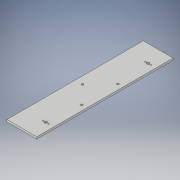
# Autodesk Inventor part: ChassisSideplate10
Saved by Autodesk Inventor 2019 (Build 230136000, 136)
## iProperties
Created: 2019-10-11
Part Number: ChassisSideplate10
Material: Generic
Document SubType Name: Modeling
Designer: shrey
Density: 1 g/cm^3
Appearance: Default
Author: shrey
Autodesk Inventor part; units mm, degrees
ref_plane "YZ Plane" through (0, 0, 0) normal (1, 0, 0) x (0, 1, 0)
ref_plane "XZ Plane" through (0, 0, 0) normal (0, 1, 0) x (-1, 0, 0)
ref_plane "XY Plane" through (0, 0, 0) normal (0, 0, 1) x (1, 0, 0)
sketch "Sketch1" plane through (0, 0, 0) normal (0, 1, 0) x (-1, 0, 0)
  line L0 (44.45, 203.2) -> (-44.45, 203.2)
  line L1 (-44.45, 203.2) -> (-44.45, -203.2)
  line L2 (-44.45, -203.2) -> (44.45, -203.2)
  line L3 (44.45, -203.2) -> (44.45, 203.2)
  line L4 (44.45, 203.2) -> (-44.45, -203.2) construction
  line L5 (-44.45, 203.2) -> (-20.955, 203.2)
  line L6 (-44.45, 88.9) -> (-44.45, 203.2)
  line L7 (44.45, 203.2) -> (44.45, 111.6492)
  line L8 (44.45, 203.2) -> (44.45, 38.1)
  line L9 (44.45, 38.1) -> (22.225, 38.1) construction
  line L10 (0, 88.9) -> (0, 203.2) construction
  line L11 (0, 203.2) -> (-66.675, 203.2)
  line L12 (-66.675, 203.2) -> (-66.675, 88.9) construction
  line L13 (-66.675, 203.2) -> (-66.675, 209.55) construction
  line L14 (-66.675, 209.55) -> (32.5679, 44.312) construction
  line L15 (-20.955, 88.9) -> (-20.955, 152.4) construction
  circle A0 centre (-20.955, 152.4) radius 8.001 construction
  circle A1 centre (-20.955, 152.4) radius 4.0005
  circle A2 centre (-20.955, 160.401) radius 1.85
  line L16 (42.545, 152.4) -> (-20.955, 152.4) construction
  circle A3 centre (-28.956, 152.4) radius 1.85
  line L17 (-20.955, 215.9) -> (-20.955, 152.4) construction
  circle A4 centre (-20.955, 144.399) radius 1.85
  line L18 (-84.455, 152.4) -> (-20.955, 152.4) construction
  circle A5 centre (-12.954, 152.4) radius 1.85
  line L19 (44.45, 0) -> (-44.45, 0) construction
  circle A6 centre (22.225, 0) radius 3.175
  circle A7 centre (-29.2932, 53.9743) radius 3.175
  line L20 (32.5679, 44.312) -> (22.7595, 60.6429) construction
  circle A8 centre (-20.955, -152.4) radius 4.0005
  circle A9 centre (-28.956, -152.4) radius 1.85
  circle A10 centre (-12.954, -152.4) radius 1.85
  circle A11 centre (-29.2932, -53.9743) radius 3.175
  point P0 (0, 0)
  point P1 (-20.955, 88.9)
  dimension "d19" = 16.002
  dimension "d0" = 88.9
  dimension "d1" = 406.4
  dimension "d5" = 165.1
  dimension "d6" = 22.225
  dimension "d10" = 6.35
  dimension "d20" = 8.001
  dimension "d21" = 3.7
  dimension "d24" = 360
  dimension "d30" = 6.35
  dimension "d31" = 6.35
  dimension "d32" = 19.05
  constraints: 42 end point, 11 centre point, 4 midpoint, 4 point on line, 4 symmetric about line, 3 horizontal, 3 parallel, 2 coincident, 1 perpendicular, 1 vertical, 1 vertical alignment, 27 other
  measures "d0" distance of L1.end L2.end
  measures "d1" distance of L0.end L1.end
  measures "d5" distance of L0.start L8.end
  measures "d6" distance of L8.end L9.end
  measures "d10" distance of L11.end L13.end
  measures "d20" diameter of A1
  measures "d21" diameter of A2
  measures "d30" diameter of A6
  measures "d31" diameter of A7
  measures "d32" distance of L14.end L20.end
extrude "Extrusion4" add sketch "Sketch1" along normal blind 6.35 contours L3 L2 L1 L0 | A2 | A4
body "Solid4"
